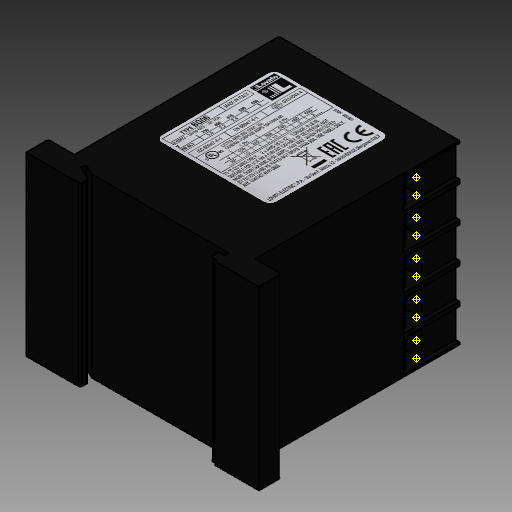
# Autodesk Inventor part: Lovato - BG0601A
Saved by Autodesk Inventor 2025.2 (Build 292293000, 293)
## iProperties
Created: 2008-01-14
Part Number: Lovato - BG0601A
Document SubType Name: Modeling
Designer: Hrvoje
Density: 1.4 g/cm^3
Material: PVC
Mass: 144.463 g
Surface Area: 194.415 cm^2
Volume: 103.188 cm^3
Appearance: Black
Description: 3-POLE RELAYS WITH AC COIL
Stock Number: 11BG0601A230
Vendor: Ellabo
OPIS: MINI SKLOPNIK BG06.01A 3P+1NC; 6A;
CIJENA: 20.5
Author: Hrvoje
Autodesk Inventor part; units mm, degrees
ref_plane "YZ Plane" through (0, 0, 0) normal (1, 0, 0) x (0, 1, 0)
ref_plane "XZ Plane" through (0, 0, 0) normal (0, 1, 0) x (-1, 0, 0)
ref_plane "XY Plane" through (0, 0, 0) normal (0, 0, 1) x (1, 0, 0)
sketch "Sketch1" plane through (0, 0, 0) normal (0, 0, 1) x (1, 0, 0)
  line L0 (0, 0.0089) -> (0, 5.0089)
  line L1 (0.5, 5.5089) -> (6.5, 5.5089)
  line L2 (6.5, 5.5089) -> (6.5, 55.5089)
  line L3 (6.5, 55.5089) -> (51.5, 55.5089)
  line L4 (51.5, 55.5089) -> (51.5, 5.5089)
  line L5 (51.5, 5.5089) -> (57.5, 5.5089)
  line L6 (58, 5.0089) -> (58, 0.0089)
  line L7 (58, 0.0089) -> (47, 0.0089)
  line L8 (47, 0.0089) -> (47, 0.5089)
  line L9 (47, 0.5089) -> (46, 0.5089)
  line L10 (45.5, 1.0089) -> (45.5, 2.0089)
  line L11 (46, 2.5089) -> (47, 2.5089)
  line L12 (47, 2.5089) -> (47, 3.5089)
  line L13 (47, 3.5089) -> (12.9082, 3.5089)
  line L14 (12.9082, 3.5089) -> (10.3819, 4.6869)
  line L15 (10.3819, 4.6869) -> (9.8748, 3.5993)
  line L16 (9.8748, 3.5993) -> (13.2113, 2.0435)
  line L17 (13.5, 1.5903) -> (13.5, 0.5089)
  line L18 (13, 0.0089) -> (0, 0.0089)
  arc A0 (46, 2.5089) -> (45.5, 2.0089) centre (46, 2.0089) ccw
  arc A1 (45.5, 1.0089) -> (46, 0.5089) centre (46, 1.0089) ccw
  arc A2 (0.5, 5.5089) -> (0, 5.0089) centre (0.5, 5.0089) ccw
  arc A3 (58, 5.0089) -> (57.5, 5.5089) centre (57.5, 5.0089) ccw
  arc A4 (13, 0.0089) -> (13.5, 0.5089) centre (13, 0.5089) ccw
  arc A5 (13.5, 1.5903) -> (13.2113, 2.0435) centre (13, 1.5903) ccw
  point P0 (0, 5.5089)
  point P1 (58, 5.5089)
  point P2 (13.5, 1.9089)
  point P3 (13.5, 0.0089)
  dimension "d0" = 58
  dimension "d1" = 6.5
  dimension "d2" = 6.5
  dimension "d4" = 5.5
  dimension "d6" = 3.5
  dimension "d7" = 13.5
  dimension "d8" = 1.9
  dimension "d9" = 1.2
  dimension "d10" = 25
  dimension "d11" = 4
  dimension "d12" = 12.5
  dimension "d13" = 11
  dimension "d14" = 1
  dimension "d15" = 0.5
  dimension "d16" = 3.5
  dimension "d17" = 0.5
  dimension "d20" = 0.5
  dimension "d21" = 55.5
  constraints: 38 end point, 12 point on circle, 12 tangent, 11 parallel, 8 point on line, 6 centre point, 5 perpendicular, 4 equal radius, 1 collinear, 1 horizontal alignment, 1 vertical, 1 vertical alignment, 1 other
  measures "d0" distance between parallel lines of L6 L0
  measures "d1" distance of point (0, 5.509) L1.end
  measures "d2" distance of L4.end point (58, 5.509)
  measures "d4" distance of L0.start point (0, 5.509)
  measures "d6" distance between parallel lines of L18 L13
  measures "d7" distance of point (13.5, 0.009) L0.start
  measures "d8" distance of point (13.5, 1.909) point (13.5, 0.009)
  measures "d9" distance of L14.end L15.end
  measures "d10" angle of L18 L16
  measures "d11" distance of L15.end point (13.5, 1.909)
  measures "d12" distance between parallel lines of L6 L10
  measures "d13" distance of L6.end L7.end
  measures "d14" distance of L11.end L12.end
  measures "d15" distance of L7.end L8.end
  measures "d16" distance between parallel lines of L7 L13
  measures "d17" radius of A0
  measures "d20" radius of A2
  measures "d21" distance between parallel lines of L18 L3
extrude "Extrusion1" add sketch "Sketch1" along normal blind 44
sketch "Sketch9" plane through (6.5, 55.5089, 0) normal (0, 1, 0) x (1, 0, 0)
  line L0 (0, -44) -> (45, -44) projected
  line L1 (45, 0) -> (45, -44) projected
  line L2 (0, 0) -> (45, 0) projected
  line L3 (0, 0) -> (0, -44) projected
  circle A0 centre (8, -13.5) radius 3
  circle A1 centre (8, -22) radius 3
  circle A2 centre (8, -30.5) radius 3
  circle A3 centre (8, -39) radius 3
  line L4 (22.5, 0) -> (22.5, -6.2339)
  circle A4 centre (37, -13.5) radius 3
  circle A5 centre (37, -22) radius 3
  circle A6 centre (37, -30.5) radius 3
  circle A7 centre (37, -39) radius 3
  circle A8 centre (7, -5) radius 3
  circle A9 centre (38, -5) radius 3
  line L5 (21, -7.5) -> (24, -7.5)
  line L6 (24, -7.5) -> (24, -16.5)
  line L7 (24, -16.5) -> (21, -16.5)
  line L8 (21, -16.5) -> (21, -7.5)
  point P0 (22.5, -7.5)
  dimension "d93" = 6
  dimension "d101" = 8.5
  dimension "d107" = 8
  dimension "d108" = 5
  dimension "d109" = 6
  dimension "d110" = 5
  dimension "d111" = 7
  dimension "d112" = 9
  dimension "d113" = 3
  dimension "d114" = 7.5
  constraints: 10 centre point, 10 end point, 5 symmetric about line, 3 parallel, 2 midpoint, 1 horizontal, 1 perpendicular, 1 vertical, 1 vertical alignment, 11 other
  measures "d93" diameter of A0
  measures "d101" distance of A0.centre A1.centre
  measures "d107" distance from line of L3 A0.centre
  measures "d108" distance from line of L0 A3.centre
  measures "d109" diameter of A8
  measures "d110" distance from line of L2 A8.centre
  measures "d111" distance from line of L3 A8.centre
  measures "d112" distance of L7.end L5.start
  measures "d113" distance of L6.end L7.end
  measures "d114" distance from line of L2 point (22.5, -7.5)
extrude "Extrusion9" add sketch "Sketch9" along normal blind 1
fillet "Fillet2" radius 0.5 1 edges at (6.5, 56.5089, 22)
sketch "Sketch10" plane through (6.5, 5.5089, 0) normal (-1, 0, 0) x (0, 0, 1)
  line L0 (0, 0) -> (0, 50.5) projected
  line L1 (44, 0) -> (44, 50.5) projected
  line L2 (44, 51) -> (0, 51) projected
  line L3 (0, 50.5) -> (0, 51) projected
  line L4 (44, 51) -> (44, 50.5) projected
  line L5 (0.95, 51) -> (8.65, 51)
  line L6 (8.65, 51) -> (8.65, 37)
  line L7 (8.65, 37) -> (0.95, 37)
  line L8 (0.95, 37) -> (0.95, 51)
  line L9 (9.55, 51) -> (17.25, 51)
  line L10 (17.25, 51) -> (17.25, 37)
  line L11 (17.25, 37) -> (9.55, 37)
  line L12 (9.55, 37) -> (9.55, 51)
  line L13 (18.15, 51) -> (25.85, 51)
  line L14 (25.85, 51) -> (25.85, 37)
  line L15 (25.85, 37) -> (18.15, 37)
  line L16 (18.15, 37) -> (18.15, 51)
  line L17 (26.75, 51) -> (34.45, 51)
  line L18 (34.45, 51) -> (34.45, 37)
  line L19 (34.45, 37) -> (26.75, 37)
  line L20 (26.75, 37) -> (26.75, 51)
  line L21 (35.35, 51) -> (43.05, 51)
  line L22 (43.05, 51) -> (43.05, 37)
  line L23 (43.05, 37) -> (35.35, 37)
  line L24 (35.35, 37) -> (35.35, 51)
  dimension "d118" = 14
  dimension "d119" = 7.7
  dimension "d120" = 0.95
  dimension "d123" = 8.6
  dimension "d128" = 0.95
  constraints: 40 end point, 2 horizontal, 2 parallel, 1 perpendicular, 1 point on line, 32 other
  measures "d118" distance of L7.end L5.start
  measures "d119" distance of L6.end L7.end
  measures "d120" distance between parallel lines of L0 L8
  measures "d123" distance of L5.start L9.start
  measures "d128" distance between parallel lines of L1 L22
extrude "Extrusion10" cut sketch "Sketch10" against normal blind 1
sketch "Sketch11" plane through (7.5, 5.5089, 0) normal (-1, 0, 0) x (0, 0, 1)
  line L0 (8.65, 37) -> (8.65, 51) projected
  line L1 (0.95, 51) -> (8.65, 51) projected
  line L2 (0.95, 51) -> (0.95, 37) projected
  line L3 (9.55, 51) -> (9.55, 37) projected
  line L4 (9.55, 37) -> (17.25, 37) projected
  line L5 (17.25, 37) -> (17.25, 51) projected
  line L6 (9.55, 51) -> (17.25, 51) projected
  line L7 (18.15, 51) -> (18.15, 37) projected
  line L8 (18.15, 37) -> (25.85, 37) projected
  line L9 (25.85, 37) -> (25.85, 51) projected
  line L10 (18.15, 51) -> (25.85, 51) projected
  line L11 (26.75, 51) -> (26.75, 37) projected
  line L12 (26.75, 37) -> (34.45, 37) projected
  line L13 (34.45, 37) -> (34.45, 51) projected
  line L14 (26.75, 51) -> (34.45, 51) projected
  line L15 (35.35, 51) -> (35.35, 37) projected
  line L16 (35.35, 37) -> (43.05, 37) projected
  line L17 (43.05, 37) -> (43.05, 51) projected
  line L18 (35.35, 51) -> (43.05, 51) projected
  line L19 (0.95, 42.5) -> (8.65, 42.5)
  line L20 (8.65, 42.5) -> (8.65, 38.5)
  line L21 (8.65, 38.5) -> (0.95, 38.5)
  line L22 (0.95, 38.5) -> (0.95, 42.5)
  line L23 (9.55, 42.5) -> (17.25, 42.5)
  line L24 (17.25, 42.5) -> (17.25, 38.5)
  line L25 (17.25, 38.5) -> (9.55, 38.5)
  line L26 (9.55, 38.5) -> (9.55, 42.5)
  line L27 (18.15, 42.5) -> (25.85, 42.5)
  line L28 (25.85, 42.5) -> (25.85, 38.5)
  line L29 (25.85, 38.5) -> (18.15, 38.5)
  line L30 (18.15, 38.5) -> (18.15, 42.5)
  line L31 (26.75, 42.5) -> (34.45, 42.5)
  line L32 (34.45, 42.5) -> (34.45, 38.5)
  line L33 (34.45, 38.5) -> (26.75, 38.5)
  line L34 (26.75, 38.5) -> (26.75, 42.5)
  line L35 (35.35, 42.5) -> (43.05, 42.5)
  line L36 (43.05, 42.5) -> (43.05, 38.5)
  line L37 (43.05, 38.5) -> (35.35, 38.5)
  line L38 (35.35, 38.5) -> (35.35, 42.5)
  dimension "d131" = 4
  dimension "d132" = 8.5
  dimension "d135" = 8.6
  constraints: 40 end point, 2 horizontal, 2 parallel, 2 point on line, 1 perpendicular, 32 other
  measures "d131" distance of L21.end L19.start
  measures "d132" distance between parallel lines of L1 L19
  measures "d135" distance of L19.end L24.start
extrude "Extrusion11" cut sketch "Sketch11" against normal blind 10 contours L21 L2 L19 L0 | L23 L5 L25 L3 | L27 L9 L29 L7 | L31 L13 L33 L11 | L35 L17 L37 L15
sketch "Sketch12" plane through (51.5, 0, 51) normal (1, 0, 0) x (0, 0, -1)
  line L0 (6.5, 56.0089) -> (51.5, 56.0089)
  line L1 (6.5, 5.5089) -> (6.5, 56.0089)
  line L2 (15.25, 56.5089) -> (15.25, 42.5089)
  line L3 (15.25, 42.5089) -> (7.55, 42.5089)
  line L4 (51, 56.5089) -> (7, 56.5089)
  line L5 (7.55, 42.5089) -> (7.55, 56.5089)
  line L6 (16.35, 42.5089) -> (16.35, 56.5089)
  line L7 (24.05, 42.5089) -> (16.35, 42.5089)
  line L8 (24.05, 56.5089) -> (24.05, 42.5089)
  line L9 (25.15, 42.5089) -> (25.15, 56.5089)
  line L10 (32.85, 42.5089) -> (25.15, 42.5089)
  line L11 (32.85, 56.5089) -> (32.85, 42.5089)
  line L12 (33.95, 42.5089) -> (33.95, 56.5089)
  line L13 (41.65, 42.5089) -> (33.95, 42.5089)
  line L14 (41.65, 56.5089) -> (41.65, 42.5089)
  line L15 (42.75, 42.5089) -> (42.75, 56.5089)
  line L16 (50.45, 42.5089) -> (42.75, 42.5089)
  line L17 (50.45, 56.5089) -> (50.45, 42.5089)
  line L18 (7.55, 56.5089) -> (15.25, 56.5089)
  line L19 (16.35, 56.5089) -> (24.05, 56.5089)
  line L20 (25.15, 56.5089) -> (32.85, 56.5089)
  line L21 (33.95, 56.5089) -> (41.65, 56.5089)
  line L22 (42.75, 56.5089) -> (50.45, 56.5089)
  dimension "d148" = 1.05
  dimension "d149" = 14
  dimension "d150" = 7.7
  dimension "d143" = 8.8
  constraints: 46 end point, 5 collinear, 2 parallel, 2 perpendicular, 2 point on line, 1 horizontal, 28 other
  measures "d148" distance between parallel lines of L1 L5
  measures "d149" distance of L3.end L5.end
  measures "d150" distance of L2.end L3.end
  measures "d143" distance of L3.end L6.start
extrude "Extrusion12" cut sketch "Sketch12" against normal blind 1 contours L5 L4 L2 L0 | L0 L2 L3 L5 | L6 L4 L8 L0 | L0 L8 L7 L6 | L9 L4 L11 L0 | L0 L11 L10 L9 | L12 L4 L14 L0 | L0 L14 L13 L12 | L15 L4 L17 L0 | L0 L17 L16 L15
sketch "Sketch13" plane through (50.5, 0, 51) normal (1, 0, 0) x (0, 0, -1)
  line L0 (7.55, 56.5089) -> (15.25, 56.5089) projected
  line L1 (7.55, 56.5089) -> (7.55, 42.5089) projected
  line L2 (15.25, 42.5089) -> (15.25, 56.5089) projected
  line L3 (24.05, 42.5089) -> (24.05, 56.5089) projected
  line L4 (16.35, 56.5089) -> (24.05, 56.5089) projected
  line L5 (16.35, 56.5089) -> (16.35, 42.5089) projected
  line L6 (16.35, 42.5089) -> (24.05, 42.5089) projected
  line L7 (32.85, 42.5089) -> (32.85, 56.5089) projected
  line L8 (25.15, 56.5089) -> (32.85, 56.5089) projected
  line L9 (25.15, 56.5089) -> (25.15, 42.5089) projected
  line L10 (25.15, 42.5089) -> (32.85, 42.5089) projected
  line L11 (41.65, 42.5089) -> (41.65, 56.5089) projected
  line L12 (33.95, 56.5089) -> (41.65, 56.5089) projected
  line L13 (33.95, 56.5089) -> (33.95, 42.5089) projected
  line L14 (33.95, 42.5089) -> (41.65, 42.5089) projected
  line L15 (50.45, 42.5089) -> (50.45, 56.5089) projected
  line L16 (42.75, 56.5089) -> (50.45, 56.5089) projected
  line L17 (42.75, 56.5089) -> (42.75, 42.5089) projected
  line L18 (42.75, 42.5089) -> (50.45, 42.5089) projected
  line L19 (7.55, 48.0089) -> (15.25, 48.0089)
  line L20 (15.25, 48.0089) -> (15.25, 44.0089)
  line L21 (15.25, 44.0089) -> (7.55, 44.0089)
  line L22 (7.55, 44.0089) -> (7.55, 48.0089)
  line L23 (16.35, 48.0089) -> (24.05, 48.0089)
  line L24 (24.05, 48.0089) -> (24.05, 44.0089)
  line L25 (24.05, 44.0089) -> (16.35, 44.0089)
  line L26 (16.35, 44.0089) -> (16.35, 48.0089)
  line L27 (25.15, 48.0089) -> (32.85, 48.0089)
  line L28 (32.85, 48.0089) -> (32.85, 44.0089)
  line L29 (32.85, 44.0089) -> (25.15, 44.0089)
  line L30 (25.15, 44.0089) -> (25.15, 48.0089)
  line L31 (33.95, 48.0089) -> (41.65, 48.0089)
  line L32 (41.65, 48.0089) -> (41.65, 44.0089)
  line L33 (41.65, 44.0089) -> (33.95, 44.0089)
  line L34 (33.95, 44.0089) -> (33.95, 48.0089)
  line L35 (42.75, 48.0089) -> (50.45, 48.0089)
  line L36 (50.45, 48.0089) -> (50.45, 44.0089)
  line L37 (50.45, 44.0089) -> (42.75, 44.0089)
  line L38 (42.75, 44.0089) -> (42.75, 48.0089)
  dimension "d154" = 4
  dimension "d155" = 8.5
  dimension "d158" = 8.8
  constraints: 40 end point, 2 horizontal, 2 parallel, 2 point on line, 1 perpendicular, 32 other
  measures "d154" distance of L21.end L19.start
  measures "d155" distance between parallel lines of L0 L19
  measures "d158" distance of L20.end L24.end
extrude "Extrusion13" cut sketch "Sketch13" against normal blind 10 contours L19 L2 L21 L1 | L25 L5 L23 L3 | L29 L9 L27 L7 | L33 L13 L31 L11 | L37 L17 L35 L15
sketch "Sketch14" plane through (6.5, 56.5089, 0) normal (0, 1, 0) x (1, 0, 0)
  circle A0 centre (8, -13.5) radius 3 projected
  circle A1 centre (8, -22) radius 3 projected
  circle A2 centre (8, -30.5) radius 3 projected
  circle A3 centre (8, -39) radius 3 projected
  circle A4 centre (37, -13.5) radius 3 projected
  circle A5 centre (37, -22) radius 3 projected
  circle A6 centre (37, -30.5) radius 3 projected
  circle A7 centre (37, -39) radius 3 projected
  circle A8 centre (7, -5) radius 3 projected
  circle A9 centre (38, -5) radius 3 projected
extrude "Extrusion14" cut sketch "Sketch14" against normal up to surface (8.5 mm away)
decal "Decal1"
sketch "Sketch16" plane through (0, 0, 44) normal (0, 0, 1) x (1, 0, 0)
  line L0 (13.0872, 18.8813) -> (13.0872, 48.8813) construction
  line L1 (13.0872, 48.8813) -> (41.9128, 48.8813) construction
  line L2 (41.9128, 48.8813) -> (41.9128, 18.8813) construction
  line L3 (41.9128, 18.8813) -> (13.0872, 18.8813) construction
  arc A0 (7, 56.5089) -> (6.5, 56.0089) centre (7, 56.0089) ccw projected
  line L4 (6.5, 5.5089) -> (6.5, 56.0089) projected
  line L5 (0.5, 5.5089) -> (6.5, 5.5089) projected
  arc A1 (0.5, 5.5089) -> (0, 5.0089) centre (0.5, 5.0089) ccw projected
  line L6 (0, 0.0089) -> (0, 5.0089) projected
  line L7 (13, 0.0089) -> (0, 0.0089) projected
  arc A2 (13, 0.0089) -> (13.5, 0.5089) centre (13, 0.5089) ccw projected
  line L8 (13.5, 1.5903) -> (13.5, 0.5089) projected
  arc A3 (13.5, 1.5903) -> (13.2113, 2.0435) centre (13, 1.5903) ccw projected
  line L9 (9.8748, 3.5993) -> (13.2113, 2.0435) projected
  line L10 (10.3819, 4.6869) -> (9.8748, 3.5993) projected
  line L11 (12.9082, 3.5089) -> (10.3819, 4.6869) projected
  line L12 (47, 3.5089) -> (12.9082, 3.5089) projected
  line L13 (47, 2.5089) -> (47, 3.5089) projected
  line L14 (46, 2.5089) -> (47, 2.5089) projected
  arc A4 (46, 2.5089) -> (45.5, 2.0089) centre (46, 2.0089) ccw projected
  line L15 (45.5, 1.0089) -> (45.5, 2.0089) projected
  arc A5 (45.5, 1.0089) -> (46, 0.5089) centre (46, 1.0089) ccw projected
  line L16 (47, 0.5089) -> (46, 0.5089) projected
  line L17 (47, 0.0089) -> (47, 0.5089) projected
  line L18 (58, 0.0089) -> (47, 0.0089) projected
  line L19 (58, 5.0089) -> (58, 0.0089) projected
  arc A6 (58, 5.0089) -> (57.5, 5.5089) centre (57.5, 5.0089) ccw projected
  line L20 (51.5, 5.5089) -> (57.5, 5.5089) projected
  line L21 (51.5, 56.5089) -> (51.5, 5.5089) projected
  line L22 (51.5, 56.5089) -> (7, 56.5089) projected
  point P0 (0, 0)
  point P1 (27.5, 48.8813)
  point P2 (27.5, 56.5089)
  dimension "d186" = 30
  constraints: 1 midpoint, 1 vertical, 1 vertical alignment, 2 other
  measures "d186" distance of L0.start L0.end
decal "Decal2"
ref_plane "Sredina" through (29, 5.5089, 44) normal (1, 0, 0) x (0, 0, -1)
sketch "Sketch17" plane through (51.5, 5.5089, 44) normal (1, 0, 0) x (0, 0, -1)
  line L0 (8.25, 51) -> (8.25, 37) construction
  line L1 (8.25, 37) -> (0.55, 37) construction
  line L2 (0.55, 37) -> (0.55, 51) construction
  line L3 (0.55, 51) -> (0, 51) construction
  line L4 (0, 51) -> (0, 0) construction
  line L5 (44, 0) -> (0, 0) construction
  line L6 (44, 51) -> (44, 0) construction
  line L7 (44, 51) -> (43.45, 51) construction
  line L8 (43.45, 51) -> (43.45, 37) construction
  line L9 (43.45, 37) -> (35.75, 37) construction
  line L10 (35.75, 37) -> (35.75, 51) construction
  line L11 (35.75, 51) -> (34.65, 51) construction
  line L12 (34.65, 51) -> (34.65, 37) construction
  line L13 (34.65, 37) -> (26.95, 37) construction
  line L14 (26.95, 37) -> (26.95, 51) construction
  line L15 (26.95, 51) -> (25.85, 51) construction
  line L16 (25.85, 51) -> (25.85, 37) construction
  line L17 (25.85, 37) -> (18.15, 37) construction
  line L18 (18.15, 37) -> (18.15, 51) construction
  line L19 (18.15, 51) -> (17.05, 51) construction
  line L20 (17.05, 51) -> (17.05, 37) construction
  line L21 (17.05, 37) -> (9.35, 37) construction
  line L22 (9.35, 37) -> (9.35, 51) construction
  line L23 (9.35, 51) -> (8.25, 51) construction
  line L24 (0.55, 42.5) -> (0.55, 38.5) construction
  line L25 (0.55, 40) -> (2.475, 40) construction
  line L26 (2.475, 40) -> (6.325, 40) construction
  line L27 (6.325, 40) -> (8.25, 40) construction
  line L28 (9.35, 40) -> (11.275, 40) construction
  line L29 (11.275, 40) -> (15.125, 40) construction
  line L30 (15.125, 40) -> (17.05, 40) construction
  line L31 (18.15, 50.5) -> (18.15, 37) construction
  line L32 (18.15, 40) -> (20.075, 40) construction
  line L33 (20.075, 40) -> (23.925, 40) construction
  line L34 (23.925, 40) -> (25.85, 40) construction
  line L35 (26.95, 40) -> (28.875, 40) construction
  line L36 (28.875, 40) -> (32.725, 40) construction
  line L37 (32.725, 40) -> (34.65, 40) construction
  line L38 (35.75, 40) -> (37.675, 40) construction
  line L39 (37.675, 40) -> (41.525, 40) construction
  line L40 (41.525, 40) -> (43.45, 40) construction
  point P0 (44, -5.5089)
  point P1 (1.5125, 40)
  dimension "d199" = 3.85
  dimension "d200" = 7.7
  dimension "d201" = 3
  constraints: 30 end point, 18 point on line, 14 collinear, 8 horizontal alignment, 3 horizontal, 2 perpendicular, 1 midpoint
  measures "d199" distance of L25.end L26.end
  measures "d200" distance of L0.end L1.end
  measures "d201" distance from line of point (1.513, 40) L1
pattern_of_nothing "Mirror1"
sketch "Sketch15" plane through (6.5, 56.5089, 0) normal (0, 1, 0) x (1, 0, 0)
  line L0 (-5.45, -44.5) -> (-5.45, 0.5) construction
  line L1 (-5.45, 0.5) -> (50.95, 0.5) construction
  line L2 (50.95, 0.5) -> (50.95, -44.5) construction
  line L3 (50.95, -44.5) -> (-5.45, -44.5) construction
  line L4 (0.5, 0) -> (45, 0) projected
  line L5 (45, -44) -> (0.5, -44) projected
  line L6 (-6, 0) -> (-6, -44) projected
  point P0 (-6.5, 0)
  point P1 (-5.45, -22)
  point P2 (-6, -22)
  point P3 (22.75, -44.5)
  point P4 (22.75, -44)
  dimension "d172" = 44
  dimension "d173" = 45
  constraints: 4 midpoint, 1 horizontal alignment, 1 vertical, 1 vertical alignment, 2 other
  measures "d172" distance between parallel lines of L4 L5
  measures "d173" distance of L0.start L0.end
equation "\"d2\" = d1"
equation "\"d109\" = d93"
equation "\"d110\" = d108"
equation "\"d199\" = 0.5 * d200"
body "Solid1"
